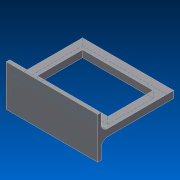
# Autodesk Inventor part: switch mount test
Saved by Autodesk Inventor 2015 (Build 190159000, 159)
## iProperties
Created: 2017-03-16
Part Number: switch mount test
Material: Generic
Document SubType Name: Modeling
Designer: ZigZagJoe
Density: 1 g/cm^3
Appearance: Default
Author: ZigZagJoe
Autodesk Inventor part; units mm, degrees
ref_plane "YZ Plane" through (0, 0, 0) normal (1, 0, 0) x (0, 1, 0)
ref_plane "XZ Plane" through (0, 0, 0) normal (0, 1, 0) x (-1, 0, 0)
ref_plane "XY Plane" through (0, 0, 0) normal (0, 0, 1) x (1, 0, 0)
sketch "Sketch1" plane through (0, 0, 0) normal (0, 0, 1) x (1, 0, 0)
  line L0 (-18.249, 5.8402) -> (8.251, 5.8402)
  line L1 (8.251, 5.8402) -> (8.251, -15.2598)
  line L2 (8.251, -15.2598) -> (-18.249, -15.2598)
  line L3 (-18.249, -15.2598) -> (-18.249, 5.8402)
  line L4 (-15.249, 2.8402) -> (5.251, 2.8402)
  line L5 (5.251, 2.8402) -> (5.251, -10.2598)
  line L6 (5.251, -10.2598) -> (-15.249, -10.2598)
  line L7 (-15.249, -10.2598) -> (-15.249, 2.8402)
  point P0 (0, 0)
  dimension "d0" = 20.5
  dimension "d1" = 13.1
  dimension "d2" = 3
  dimension "d3" = 3
  dimension "d4" = 5
  dimension "d5" = 3
  constraints: 16 end point, 4 parallel, 2 horizontal, 2 perpendicular
  measures "d0" distance of L5.end L6.end
  measures "d1" distance of L4.end L5.end
  measures "d2" distance between parallel lines of L4 L0
  measures "d3" distance between parallel lines of L1 L5
  measures "d4" distance between parallel lines of L2 L6
  measures "d5" distance between parallel lines of L3 L7
extrude "Extrusion1" add sketch "Sketch1" along normal blind 2
sketch "Sketch2" plane through (-18.249, -15.2598, 0) normal (0, -1, 0) x (1, 0, 0)
  line L0 (-0.0474, 7) -> (26.5, 7)
  line L1 (26.5, 7) -> (26.5, -5)
  line L2 (26.5, -5) -> (-0.0474, -5)
  line L3 (-0.0474, -5) -> (-0.0474, 7)
  line L4 (0, 2) -> (26.5, 2) projected
  line L5 (26.5, 0) -> (0, 0) projected
  line L6 (26.5, 0) -> (26.5, 2) projected
  point P0 (18.249, 0)
  dimension "d8" = 5
  dimension "d9" = 5
  dimension "d10" = 0
  constraints: 8 end point, 2 parallel, 1 horizontal, 1 perpendicular
  measures "d8" distance between parallel lines of L0 L4
  measures "d9" distance between parallel lines of L2 L5
  measures "d10" distance between parallel lines of L6 L1
extrude "Extrusion2" add sketch "Sketch2" along normal blind 1
fillet "Fillet1" radius 2 2 edges at (-4.999, -15.2598, 2) (-4.999, -15.2598, 0)
body "Solid1"
